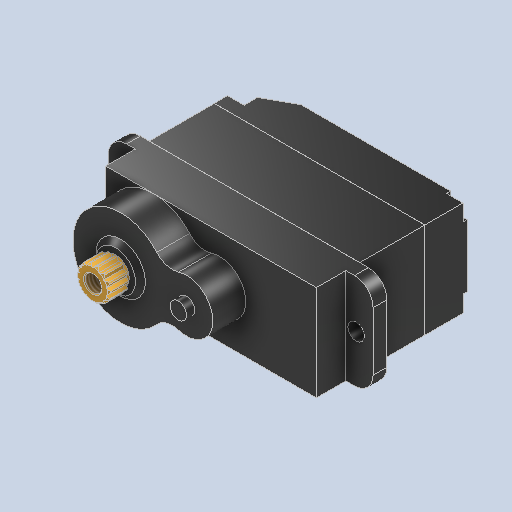
# Autodesk Inventor part: Servo EMAX ES08MDII
Saved by Autodesk Inventor 2023 (Build 270158000, 158)
## iProperties
Created: 2024-10-05
Part Number: Servo EMAX ES08MDII
Material: Generic
Document SubType Name: Modeling
Designer: akhsanu
Density: 1 g/cm^3
Appearance: Glossy - Black
Author: akhsanu
Autodesk Inventor part; units mm, degrees
ref_plane "YZ Plane" through (0, 0, 0) normal (1, 0, 0) x (0, 1, 0)
ref_plane "XZ Plane" through (0, 0, 0) normal (0, 1, 0) x (-1, 0, 0)
sketch "Sketch1" plane through (0, 0, 0) normal (0, 0, 1) x (1, 0, 0)
  line L0 (-5.79, 5.79) -> (19.75, 5.79)
  line L1 (19.75, 5.79) -> (19.75, -5.79)
  line L2 (19.75, -5.79) -> (-5.79, -5.79)
  line L3 (-5.79, -5.79) -> (-5.79, 5.79)
  arc A0 (4.3739, 3.7938) -> (4.3739, -3.7938) centre (0, 0) ccw
  arc A1 (7.0202, -3.0495) -> (7.0202, 3.0495) centre (7.99, 0) ccw
  arc A2 (7.0202, -3.0495) -> (4.3739, -3.7938) centre (6.2625, -5.4319) ccw
  arc A3 (4.3739, 3.7938) -> (7.0202, 3.0495) centre (6.2625, 5.4319) ccw
  line L4 (-5.79, 5.79) -> (-6.84, 5.79)
  line L5 (-9.09, 3.54) -> (-9.09, -3.54)
  line L6 (-6.84, -5.79) -> (-5.79, -5.79)
  line L7 (19.75, 5.79) -> (20.8, 5.79)
  line L8 (23.05, 3.54) -> (23.05, -3.54)
  line L9 (20.8, -5.79) -> (19.75, -5.79)
  circle A4 centre (-7.02, 0) radius 1
  circle A5 centre (20.98, 0) radius 1
  arc A6 (-6.84, 5.79) -> (-9.09, 3.54) centre (-6.84, 3.54) ccw
  arc A7 (-9.09, -3.54) -> (-6.84, -5.79) centre (-6.84, -3.54) ccw
  arc A8 (20.8, -5.79) -> (23.05, -3.54) centre (20.8, -3.54) ccw
  arc A9 (23.05, 3.54) -> (20.8, 5.79) centre (20.8, 3.54) ccw
  point P0 (23.05, 5.79)
  point P1 (23.05, -5.79)
  point P2 (6.98, 5.79)
  dimension "d0" = 25.54
  dimension "d1" = 11.58
  dimension "d2" = 11.58
  dimension "d3" = 6.4
  dimension "d4" = 8.56
  dimension "d5" = 5
  dimension "d6" = 5
  dimension "d7" = 32.14
  dimension "d8" = 16.07
  dimension "d9" = 2
  dimension "d10" = 2
  dimension "d11" = 28
  dimension "d12" = 14
  dimension "d13" = 2.25
  constraints: 20 end point, 16 point on circle, 14 tangent, 10 centre point, 6 point on line, 5 perpendicular, 3 equal radius, 3 horizontal alignment, 2 horizontal, 2 parallel, 1 coincident, 1 midpoint
  measures "d0" distance of L1.end L2.end
  measures "d1" distance of L0.end L1.end
  measures "d2" diameter of A0
  measures "d3" diameter of A1
  measures "d4" distance edge to line of A1 L1
  measures "d5" diameter of A2
  measures "d6" diameter of A3
  measures "d7" distance between parallel lines of L5 L8
  measures "d8" distance from line of point (6.98, 5.79) L5
  measures "d9" diameter of A4
  measures "d10" diameter of A5
  measures "d11" distance of A5.centre A4.centre
  measures "d12" horizontal distance of point (6.98, 5.79) A4.centre
  measures "d13" radius of A6
extrude "Extrusion1" add sketch "Sketch1" along normal blind 3.58 contours L0 A0 L3 | L0 L1 L2 A0 A2 A1 A3 | A0 A3 A1 A2 | A0 L2 L3
extrude "Extrusion2" add sketch "Sketch1" along normal blind 7.56 contours A0 A3 A1 A2
extrude "Extrusion3" add sketch "Sketch1" against normal blind 1.68
extrude "Extrusion4" add sketch "Sketch1" against normal blind 14.7 contours L0 A0 L3 | L0 L1 L2 A0 A2 A1 A3 | A0 A3 A1 A2 | A0 L2 L3
sketch "Sketch2" plane through (0, 0, 7.56) normal (0, 0, 1) x (1, 0, 0)
  circle A0 centre (0, 0) radius 3
  circle A1 centre (0, 0) radius 2
  arc A2 (7.0202, -3.0495) -> (7.0202, 3.0495) centre (7.99, 0) ccw projected
  arc A3 (7.0202, -3.0495) -> (4.3739, -3.7938) centre (6.2625, -5.4319) ccw projected
  arc A4 (4.3739, 3.7938) -> (4.3739, -3.7938) centre (0, 0) ccw projected
  arc A5 (4.3739, 3.7938) -> (7.0202, 3.0495) centre (6.2625, 5.4319) ccw projected
  circle A6 centre (7.99, 0) radius 1
  dimension "d22" = 6
  dimension "d23" = 4
  dimension "d24" = 2
  constraints: 3 centre point, 3 coincident
  measures "d22" diameter of A0
  measures "d23" diameter of A1
  measures "d24" diameter of A6
extrude "Extrusion5" add sketch "Sketch2" along normal blind 0.6 contours A0 | A1
extrude "Extrusion6" add sketch "Sketch2" along normal blind 3.4 contours A1
extrude "Extrusion7" add sketch "Sketch2" along normal blind 1 contours A6
chamfer "Chamfer1" distance 0.6 angle 45 1 edges at (-3, 0, 8.16)
sketch "Sketch3" plane through (0, 0, -1.68) normal (0, 0, -1) x (-1, 0, 0)
  circle A0 centre (-20.98, 0) radius 1 projected
  circle A1 centre (7.02, 0) radius 1 projected
  arc A2 (9.09, 3.54) -> (6.84, 5.79) centre (6.84, 3.54) ccw projected
  line L0 (9.09, 3.54) -> (9.09, -3.54) projected
  arc A3 (6.84, -5.79) -> (9.09, -3.54) centre (6.84, -3.54) ccw projected
  line L1 (6.84, -5.79) -> (5.79, -5.79) projected
  line L2 (5.79, 5.79) -> (5.79, -5.79) projected
  line L3 (-19.75, 5.79) -> (5.79, 5.79) projected
  line L4 (-19.75, -5.79) -> (-19.75, 5.79) projected
  line L5 (-19.75, -5.79) -> (-20.8, -5.79) projected
  arc A4 (-23.05, -3.54) -> (-20.8, -5.79) centre (-20.8, -3.54) ccw projected
  line L6 (-23.05, -3.54) -> (-23.05, 3.54) projected
  arc A5 (-20.8, 5.79) -> (-23.05, 3.54) centre (-20.8, 3.54) ccw projected
  line L7 (-20.8, 5.79) -> (-19.75, 5.79) projected
  line L8 (5.79, 5.79) -> (6.84, 5.79) projected
  line L9 (5.79, -5.79) -> (-19.75, -5.79) projected
  line L10 (-19.74, -5.78) -> (-19.74, 5.78)
  line L11 (5.78, 5.78) -> (5.78, -5.78)
  line L12 (-19.74, 5.78) -> (5.78, 5.78)
  line L13 (5.78, -5.78) -> (-19.74, -5.78)
  point P0 (0, 0)
  dimension "d37" = 0.01
  dimension "d38" = 0.01
  dimension "d39" = 0.01
  dimension "d40" = 0.01
  constraints: 8 end point, 4 parallel
  measures "d37" distance between parallel lines of L4 L10
  measures "d38" distance between parallel lines of L2 L11
  measures "d39" distance between parallel lines of L3 L12
  measures "d40" distance between parallel lines of L9 L13
extrude "Extrusion8" cut sketch "Sketch3" along normal blind 7.9 contours L2 L9 L4 L3
chamfer "Chamfer3" distance 5.4 distance2 3 1 edges at (-5.79, 0, -14.7) measured on face at (11.2367, -1.93, -14.7)
sketch "Sketch4" plane through (0, 0, -14.7) normal (0, 0, -1) x (-1, 0, 0)
  line L0 (0.39, 5.79) -> (0.39, -5.79) projected
  line L1 (0.39, -5.79) -> (-19.75, -5.79) projected
  line L2 (-19.75, -5.79) -> (-19.75, 5.79) projected
  line L3 (-19.75, 5.79) -> (0.39, 5.79) projected
  line L4 (5.79, -5.79) -> (5.79, 5.79) projected
  line L5 (0.39, -5.79) -> (5.79, -5.79) projected
  line L6 (5.79, 5.79) -> (0.39, 5.79) projected
  line L7 (5.79, -5.79) -> (3.79, -5.79)
  line L8 (3.79, -5.79) -> (3.79, -4.79)
  line L9 (4.79, -3.79) -> (5.79, -3.79)
  line L10 (5.79, -3.79) -> (5.79, -5.79)
  line L11 (5.79, 5.79) -> (3.79, 5.79)
  line L12 (3.79, 5.79) -> (3.79, 4.79)
  line L13 (4.79, 3.79) -> (5.79, 3.79)
  line L14 (5.79, 3.79) -> (5.79, 5.79)
  arc A0 (4.79, -3.79) -> (3.79, -4.79) centre (4.79, -4.79) ccw
  arc A1 (3.79, 4.79) -> (4.79, 3.79) centre (4.79, 4.79) ccw
  line L15 (-19.75, -5.79) -> (-17.75, -5.79)
  line L16 (-17.75, -5.79) -> (-17.75, -4.79)
  line L17 (-18.75, -3.79) -> (-19.75, -3.79)
  line L18 (-19.75, -3.79) -> (-19.75, -5.79)
  line L19 (-19.75, 5.79) -> (-17.75, 5.79)
  line L20 (-17.75, 5.79) -> (-17.75, 4.79)
  line L21 (-18.75, 3.79) -> (-19.75, 3.79)
  line L22 (-19.75, 3.79) -> (-19.75, 5.79)
  arc A2 (-18.75, 3.79) -> (-17.75, 4.79) centre (-18.75, 4.79) ccw
  arc A3 (-17.75, -4.79) -> (-18.75, -3.79) centre (-18.75, -4.79) ccw
  line L23 (5.79, 5.79) -> (5.79, -5.79) projected
  line L24 (5.79, 2) -> (4.79, 2)
  line L25 (4.79, 2) -> (4.79, -2)
  line L26 (4.79, -2) -> (5.79, -2)
  line L27 (5.79, -2) -> (5.79, 2)
  line L28 (4.8, 1.99) -> (5.78, 1.99)
  line L29 (5.78, 1.99) -> (5.78, -1.99)
  line L30 (5.78, -1.99) -> (4.8, -1.99)
  line L31 (4.8, -1.99) -> (4.8, 1.99)
  line L32 (5.78, 1.99) -> (5.79, 1.99)
  line L33 (5.78, -1.99) -> (5.79, -1.99)
  point P0 (0, 0)
  point P1 (3.79, -3.79)
  point P2 (3.79, 3.79)
  point P3 (-19.74, -5.78)
  point P4 (-19.74, 5.78)
  point P5 (-17.75, -3.79)
  point P6 (-17.75, 3.79)
  point P7 (4.79, 0)
  point P8 (5.79, 0)
  dimension "d46" = 2
  dimension "d47" = 2
  dimension "d48" = 2
  dimension "d49" = 2
  dimension "d54" = 1
  dimension "d55" = 2
  dimension "d56" = 2
  dimension "d57" = 2
  dimension "d58" = 2
  dimension "d59" = 1
  dimension "d97" = 1
  dimension "d98" = 4
  dimension "d99" = 0.01
  constraints: 52 end point, 12 parallel, 11 point on line, 8 point on circle, 8 tangent, 7 perpendicular, 6 horizontal, 4 centre point, 2 equal radius, 2 midpoint, 1 horizontal alignment, 3 other
  measures "d46" distance of point (3.79, -3.79) L9.end
  measures "d47" distance of L7.end point (3.79, -3.79)
  measures "d48" distance of L13.end point (3.79, 3.79)
  measures "d49" distance of point (3.79, 3.79) L11.end
  measures "d54" radius of A0
  measures "d55" distance of L17.end point (-17.75, -3.79)
  measures "d56" distance of point (-17.75, -3.79) L15.end
  measures "d57" distance of point (-17.75, 3.79) L21.end
  measures "d58" distance of L19.end point (-17.75, 3.79)
  measures "d59" radius of A2
  measures "d97" distance of L26.end L25.end
  measures "d98" distance of L25.end L24.end
  measures "d99" distance between parallel lines of L24 L28
extrude "Extrusion9" cut sketch "Sketch4" against normal blind 3.5 contours L6 L4 L13 A1 L12 | L8 A0 L9 L4 L5
extrude "Extrusion10" cut sketch "Sketch4" against normal blind 0.5 contours L20 A2 L21 L2 L3 | L1 L2 L17 A3 L16
chamfer "Chamfer4" distance 0.2 angle 45 1 edges at (-2, 0, 10.96)
sketch "Sketch5" plane through (0, 0, 10.96) normal (0, 0, 1) x (1, 0, 0)
  circle A0 centre (0, 0) radius 2 projected
  line L0 (-0.35, 1.9691) -> (0, 1.7)
  line L1 (0, 1.7) -> (0.35, 1.9691)
  line L2 (-1.1697, 1.6223) -> (-0.7376, 1.5316)
  line L3 (-0.7376, 1.5316) -> (-0.539, 1.926)
  line L4 (-1.7578, 0.9541) -> (-1.3291, 1.0599)
  line L5 (-1.3291, 1.0599) -> (-1.3213, 1.5014)
  line L6 (-1.9976, 0.0969) -> (-1.6574, 0.3783)
  line L7 (-1.6574, 0.3783) -> (-1.8419, 0.7794)
  line L8 (-1.8419, -0.7794) -> (-1.6574, -0.3783)
  line L9 (-1.6574, -0.3783) -> (-1.9976, -0.0969)
  line L10 (-1.3213, -1.5014) -> (-1.3291, -1.0599)
  line L11 (-1.3291, -1.0599) -> (-1.7578, -0.9541)
  line L12 (-0.539, -1.926) -> (-0.7376, -1.5316)
  line L13 (-0.7376, -1.5316) -> (-1.1697, -1.6223)
  line L14 (0.35, -1.9691) -> (0, -1.7)
  line L15 (0, -1.7) -> (-0.35, -1.9691)
  line L16 (1.1697, -1.6223) -> (0.7376, -1.5316)
  line L17 (0.7376, -1.5316) -> (0.539, -1.926)
  line L18 (1.7578, -0.9541) -> (1.3291, -1.0599)
  line L19 (1.3291, -1.0599) -> (1.3213, -1.5014)
  line L20 (1.9976, -0.0969) -> (1.6574, -0.3783)
  line L21 (1.6574, -0.3783) -> (1.8419, -0.7794)
  line L22 (1.8419, 0.7794) -> (1.6574, 0.3783)
  line L23 (1.6574, 0.3783) -> (1.9976, 0.0969)
  line L24 (1.3213, 1.5014) -> (1.3291, 1.0599)
  line L25 (1.3291, 1.0599) -> (1.7578, 0.9541)
  line L26 (0.539, 1.926) -> (0.7376, 1.5316)
  line L27 (0.7376, 1.5316) -> (1.1697, 1.6223)
  circle A1 centre (0, 0) radius 1.8 projected
  dimension "d64" = 0.7
  dimension "d65" = 0.35
  dimension "d66" = 1.7
  dimension "d69" = 360
  constraints: 56 end point, 2 point on circle, 1 vertical alignment, 71 other
  measures "d64" distance of L1.end L0.start
  measures "d65" horizontal distance of point (0, 0) L0.start
  measures "d66" distance of point (0, 0) L0.end
extrude "Extrusion12" cut sketch "Sketch5" against normal up to surface (2.8 mm away) contours L1 A1 L0 A0 | L1 L0 A1
pattern_circular "Circular Pattern2" count 14 over 360 about axis through (0, 0, 7.56) along (0, 0, 1) of "Extrusion12"
ref_plane "Work Plane1" through (0, 0, 8.56) normal (0, 0, 1) x (1, 0, 0)
sketch "Sketch6" plane through (0, 0, 8.56) normal (0, 0, 1) x (1, 0, 0)
  line L0 (0, 1.7) -> (0.35, 1.9691) projected
  arc A0 (0.539, 1.926) -> (0.35, 1.9691) centre (0, 0) ccw projected
  line L1 (0.539, 1.926) -> (0.7376, 1.5316) projected
  line L2 (0.7376, 1.5316) -> (1.1697, 1.6223) projected
  arc A1 (1.3213, 1.5014) -> (1.1697, 1.6223) centre (0, 0) ccw projected
  line L3 (1.3213, 1.5014) -> (1.3291, 1.0599) projected
  line L4 (1.3291, 1.0599) -> (1.7578, 0.9541) projected
  arc A2 (1.8419, 0.7794) -> (1.7578, 0.9541) centre (0, 0) ccw projected
  line L5 (1.8419, 0.7794) -> (1.6574, 0.3783) projected
  line L6 (1.6574, 0.3783) -> (1.9976, 0.0969) projected
  arc A3 (1.9976, -0.0969) -> (1.9976, 0.0969) centre (0, 0) ccw projected
  line L7 (1.9976, -0.0969) -> (1.6574, -0.3783) projected
  line L8 (1.6574, -0.3783) -> (1.8419, -0.7794) projected
  arc A4 (1.7578, -0.9541) -> (1.8419, -0.7794) centre (0, 0) ccw projected
  line L9 (1.7578, -0.9541) -> (1.3291, -1.0599) projected
  line L10 (1.3291, -1.0599) -> (1.3213, -1.5014) projected
  arc A5 (1.1697, -1.6223) -> (1.3213, -1.5014) centre (0, 0) ccw projected
  line L11 (1.1697, -1.6223) -> (0.7376, -1.5316) projected
  line L12 (0.7376, -1.5316) -> (0.539, -1.926) projected
  arc A6 (0.35, -1.9691) -> (0.539, -1.926) centre (0, 0) ccw projected
  line L13 (0.35, -1.9691) -> (0, -1.7) projected
  line L14 (0, -1.7) -> (-0.35, -1.9691) projected
  arc A7 (-0.539, -1.926) -> (-0.35, -1.9691) centre (0, 0) ccw projected
  line L15 (-0.539, -1.926) -> (-0.7376, -1.5316) projected
  line L16 (-0.7376, -1.5316) -> (-1.1697, -1.6223) projected
  arc A8 (-1.3213, -1.5014) -> (-1.1697, -1.6223) centre (0, 0) ccw projected
  line L17 (-1.3213, -1.5014) -> (-1.3291, -1.0599) projected
  line L18 (-1.3291, -1.0599) -> (-1.7578, -0.9541) projected
  arc A9 (-1.8419, -0.7794) -> (-1.7578, -0.9541) centre (0, 0) ccw projected
  line L19 (-1.8419, -0.7794) -> (-1.6574, -0.3783) projected
  line L20 (-1.6574, -0.3783) -> (-1.9976, -0.0969) projected
  arc A10 (-1.9976, 0.0969) -> (-1.9976, -0.0969) centre (0, 0) ccw projected
  line L21 (-1.9976, 0.0969) -> (-1.6574, 0.3783) projected
  line L22 (-1.6574, 0.3783) -> (-1.8419, 0.7794) projected
  arc A11 (-1.7578, 0.9541) -> (-1.8419, 0.7794) centre (0, 0) ccw projected
  line L23 (-1.7578, 0.9541) -> (-1.3291, 1.0599) projected
  line L24 (-1.3291, 1.0599) -> (-1.3213, 1.5014) projected
  arc A12 (-1.1697, 1.6223) -> (-1.3213, 1.5014) centre (0, 0) ccw projected
  line L25 (-1.1697, 1.6223) -> (-0.7376, 1.5316) projected
  line L26 (-0.7376, 1.5316) -> (-0.539, 1.926) projected
  arc A13 (-0.35, 1.9691) -> (-0.539, 1.926) centre (0, 0) ccw projected
  line L27 (-0.35, 1.9691) -> (0, 1.7) projected
  circle A14 centre (7.99, 0) radius 1 projected
  circle A15 centre (0, 0) radius 1.65
  dimension "d85" = 3.3
  constraints: 1 centre point, 1 coincident
  measures "d85" diameter of A15
extrude "Extrusion13" cut sketch "Sketch6" against normal up to surface (0.4 mm away) contours L0 A0 L1 L2 A1 L3 L4 A2 L5 L6 A3 L7 L8 A4 L9 L10 A5 L11 L12 A6 L13 L14 A7 L15 L16 A8 L17 L18 A9 L19 L20 A10 L21 L22 A11 L23 L24 A12 L25 L26 A13 L27
sketch "Sketch7" plane through (0, 0, 10.96) normal (0, 0, 1) x (1, 0, 0)
  arc A0 (0.667, 1.6719) -> (0.1244, 1.7957) centre (0, 0) ccw projected
  constraints: 1 coincident
hole "Hole1" at (0, 0, 10.96) direction (0, 0, -1) diameter 2 depth 5 countersink diameter 2.2 countersink angle 90
thread "Thread1" size "M2x0.4" class "6H" standard "ANSI Metric M Profile" full length
extrude "Extrusion14" cut sketch "Sketch4" against normal blind 4.5 contours L4 L32 L28 L31 L30 L33 L26 L25 L24 | L29 L30 L31 L28
equation "\"d6\" = d5"
equation "\"d8\" = 0.5 * d7"
equation "\"d12\" = 0.5 * d11"
equation "\"d38\" = d39"
equation "\"d39\" = d40"
equation "\"d40\" = d37"
equation "\"d65\" = 0.5 * d64"
body "Solid1"
